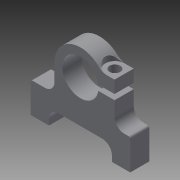
# Autodesk Inventor part: 535638-12mmClampingBracket
Saved by Autodesk Inventor 2013 (Build 170138000, 138)
## iProperties
Created: 2015-04-26
Part Number: 535638-12mmClampingBracket
Material: Generic
Document SubType Name: Modeling
Designer: Excalibur
Density: 1 g/cm^3
Author: Excalibur
Autodesk Inventor part; units mm, degrees
ref_plane "YZ Plane" through (0, 0, 0) normal (1, 0, 0) x (0, 1, 0)
ref_plane "XZ Plane" through (0, 0, 0) normal (0, 1, 0) x (-1, 0, 0)
ref_plane "XY Plane" through (0, 0, 0) normal (0, 0, 1) x (1, 0, 0)
sketch "Sketch1" plane through (0, 0, 0) normal (0, 0, 1) x (1, 0, 0)
  line L0 (0, 0) -> (0, 14.864) construction
  arc A0 (0, 25.05) -> (0, 13.05) centre (0, 19.05) ccw
  line L1 (-10.4394, 0) -> (-10.4394, 1.905)
  line L2 (-7.2644, 5.08) -> (0, 5.08)
  line L3 (-16.51, 0) -> (-16.51, 9.525)
  line L4 (-15.875, 10.16) -> (-11.811, 10.16)
  line L5 (-8.636, 13.335) -> (-8.636, 19.05)
  arc A1 (0, 27.686) -> (-8.636, 19.05) centre (0, 19.05) ccw
  arc A2 (-7.2644, 5.08) -> (-10.4394, 1.905) centre (-7.2644, 1.905) ccw
  line L6 (-10.4394, 0) -> (-16.51, 0)
  arc A3 (-15.875, 10.16) -> (-16.51, 9.525) centre (-15.875, 9.525) ccw
  arc A4 (-11.811, 10.16) -> (-8.636, 13.335) centre (-11.811, 13.335) ccw
  arc A5 (5.9338, 19.939) -> (0, 25.05) centre (0, 19.05) ccw
  arc A6 (0, 13.05) -> (5.9338, 18.161) centre (0, 19.05) ccw
  arc A7 (6.0886, 25.1745) -> (0, 27.686) centre (0, 19.05) ccw
  line L7 (8.7747, 24.0665) -> (11.3186, 24.0665)
  line L8 (11.3186, 24.0665) -> (11.3186, 19.939)
  line L9 (11.3186, 19.939) -> (5.9338, 19.939)
  line L10 (5.9338, 18.161) -> (11.3186, 18.161)
  line L11 (11.3186, 18.161) -> (11.3186, 13.335)
  line L12 (14.4936, 10.16) -> (15.875, 10.16)
  line L13 (16.51, 9.525) -> (16.51, 0)
  line L14 (16.51, 0) -> (10.4394, 0)
  line L15 (10.4394, 0) -> (10.4394, 1.905)
  line L16 (7.2644, 5.08) -> (0, 5.08)
  arc A8 (10.4394, 1.905) -> (7.2644, 5.08) centre (7.2644, 1.905) ccw
  arc A9 (11.3186, 13.335) -> (14.4936, 10.16) centre (14.4936, 13.335) ccw
  arc A10 (16.51, 9.525) -> (15.875, 10.16) centre (15.875, 9.525) ccw
  line L17 (0, 19.05) -> (12.673, 19.05) construction
  arc A11 (6.0886, 25.1745) -> (8.7747, 24.0665) centre (8.7747, 27.8765) ccw
  point P0 (7.0296, 24.0665)
  dimension "d0" = 19.05
  dimension "d1" = 6
  dimension "d2" = 27.686
  dimension "d3" = 3.175
  dimension "d4" = 0.635
  dimension "d5" = 3.175
  dimension "d6" = 33.02
  dimension "d7" = 10.16
  dimension "d8" = 6.0706
  dimension "d9" = 5.08
  dimension "d10" = 3.175
  dimension "d11" = 0.635
  dimension "d12" = 5.3848
  dimension "d13" = 1.778
  dimension "d14" = 3.81
  dimension "d15" = 4.1275
  constraints: 36 end point, 25 point on circle, 18 tangent, 12 centre point, 10 parallel, 7 point on line, 6 collinear, 6 perpendicular, 3 coincident, 1 concentric, 1 equal radius, 1 vertical, 1 other
  measures "d0" distance of L0.start A0.centre
  measures "d1" radius of A0
  measures "d2" distance of L0.start A1.start
  measures "d3" radius of A2
  measures "d4" radius of A3
  measures "d5" radius of A4
  measures "d6" diameter of L3 L0
  measures "d7" distance between parallel lines of L6 L4
  measures "d8" distance of L1.start L3.start
  measures "d9" distance between parallel lines of L6 L2
  measures "d10" radius of A8
  measures "d11" radius of A10
  measures "d12" distance of L10.start L10.end
  measures "d13" distance between parallel lines of L10 L9
  measures "d14" radius of A11
  measures "d15" distance of L7.end L8.end
extrude "Extrusion1" add sketch "Sketch1" along normal blind 6.35
sketch "Sketch3" plane through (8.7747, 24.0665, 0) normal (0, 1, 0) x (1, 0, 0)
  line L0 (0, 0) -> (2.5438, 0) projected
  line L1 (2.5438, -6.35) -> (0, -6.35) projected
  line L2 (2.5438, 0) -> (2.5438, -6.35) projected
  line L3 (2.5438, -3.175) -> (-0.5042, -3.175) construction
  line L4 (0, 0) -> (-0.5042, 0)
  line L5 (0, -6.35) -> (-0.5042, -6.35)
  arc A0 (-0.5042, 0) -> (-0.5042, -6.35) centre (-0.5042, -3.175) ccw
  point P0 (-8.7747, 0)
  dimension "d22" = 3.048
  constraints: 6 end point, 2 parallel, 2 point on circle, 2 tangent, 1 centre point, 1 coincident, 1 midpoint, 1 perpendicular
  measures "d22" distance of L3.start L3.end
extrude "Extrusion2" cut sketch "Sketch3" along normal blind 6.35
sketch "Sketch4" plane through (11.3186, 24.0665, 6.35) normal (0, 1, 0) x (1, 0, 0)
  arc A0 (-3.048, 6.35) -> (-3.048, 0) centre (-3.048, 3.175) ccw projected
  point P0 (-11.3186, 6.35)
hole "Hole1" at (8.2706, 24.0665, 3.175) direction (0, -1, 0) diameter 3.556 depth 5.08
sketch "Sketch5" plane through (5.9338, 18.161, 0) normal (0, 1, 0) x (1, 0, 0)
  circle A0 centre (2.3368, -3.175) radius 1.778 projected
  point P0 (-5.9338, 0)
hole "Hole2" at (8.2706, 18.161, 3.175) direction (0, -1, 0) diameter 2.6416 depth 6.35 tip angle 118 thread size "6-32 UNC" class "2B" standard "ANSI Unified Screw Threads"
sketch "Sketch6" plane through (-16.51, 0, 0) normal (0, -1, 0) x (1, 0, 0)
  line L0 (33.02, 0) -> (26.9494, 0) projected
  line L1 (33.02, 0) -> (33.02, 6.35) projected
  line L2 (26.9494, 6.35) -> (33.02, 6.35) projected
  line L3 (26.9494, 0) -> (26.9494, 6.35) projected
  line L4 (0, 0) -> (6.0706, 6.35) construction
  line L5 (26.9494, 0) -> (33.02, 6.35) construction
  point P0 (16.51, 0)
  point P1 (3.0353, 3.175)
  point P2 (29.9847, 3.175)
  constraints: 4 end point, 2 midpoint, 1 parallel
hole "Hole3" at (-13.4747, 0, 3.175) at (13.4747, 0, 3.175) direction (0, 1, 0) diameter 2.6416 depth 8.89 tip angle 118 thread size "6-32 UNC" class "2B" standard "ANSI Unified Screw Threads"
body "Solid1"
